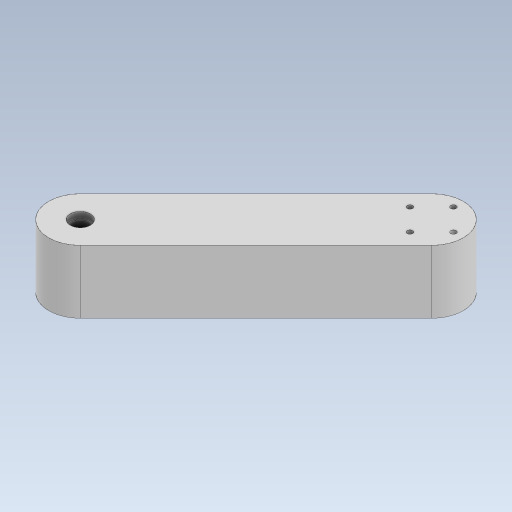
# Autodesk Inventor part: 5 Barras Simplificado
Saved by Autodesk Inventor 2024.2 (Build 282272000, 272)
## iProperties
Created: 2024-02-01
Part Number: 5 Barras Simplificado
Material: Generic
Document SubType Name: Modeling
Designer: juanp
Density: 1 g/cm^3
Appearance: Default
Author: juanp
Autodesk Inventor part; units mm, degrees
ref_plane "YZ Plane" through (0, 0, 0) normal (1, 0, 0) x (0, 1, 0)
ref_plane "XZ Plane" through (0, 0, 0) normal (0, 1, 0) x (-1, 0, 0)
ref_plane "XY Plane" through (0, 0, 0) normal (0, 0, 1) x (1, 0, 0)
sketch "Sketch1" plane through (0, 0, 0) normal (0, 1, 0) x (-1, 0, 0)
  line L0 (1000, 500) -> (0, 500) construction
  line L1 (0, 500) -> (0, -500) construction
  line L2 (0, -500) -> (1000, -500) construction
  line L3 (1000, -500) -> (1000, 500) construction
  line L4 (0, 75) -> (0, -75) construction
  line L5 (25.4, 75) -> (25.4, -75)
  line L6 (-25.4, -75) -> (-25.4, 75)
  arc A0 (25.4, 75) -> (-25.4, 75) centre (0, 75) ccw
  arc A1 (-25.4, -75) -> (25.4, -75) centre (0, -75) ccw
  line L7 (141.4214, 216.4214) -> (0, 75) construction
  line L8 (123.4608, 234.3819) -> (-17.9605, 92.9605)
  line L9 (17.9605, 57.0395) -> (159.3819, 198.4608)
  arc A2 (159.3819, 198.4608) -> (123.4608, 234.3819) centre (141.4214, 216.4214) ccw
  arc A3 (-17.9605, 92.9605) -> (17.9605, 57.0395) centre (0, 75) ccw
  line L10 (141.4214, -216.4214) -> (0, -75) construction
  line L11 (159.3819, -198.4608) -> (17.9605, -57.0395)
  line L12 (-17.9605, -92.9605) -> (123.4608, -234.3819)
  arc A4 (123.4608, -234.3819) -> (159.3819, -198.4608) centre (141.4214, -216.4214) ccw
  arc A5 (17.9605, -57.0395) -> (-17.9605, -92.9605) centre (0, -75) ccw
  line L13 (141.4214, 216.4214) -> (477.8167, 0) construction
  line L14 (155.1641, 237.7825) -> (491.5594, 21.3611)
  line L15 (464.0739, -21.3611) -> (127.6786, 195.0603)
  arc A6 (155.1641, 237.7825) -> (127.6786, 195.0603) centre (141.4214, 216.4214) ccw
  arc A7 (464.0739, -21.3611) -> (491.5594, 21.3611) centre (477.8167, 0) ccw
  line L16 (141.4214, -216.4214) -> (477.8167, 0) construction
  line L17 (155.1641, -237.7825) -> (491.5594, -21.3611)
  line L18 (464.0739, 21.3611) -> (127.6786, -195.0603)
  arc A8 (127.6786, -195.0603) -> (155.1641, -237.7825) centre (141.4214, -216.4214) ccw
  arc A9 (491.5594, -21.3611) -> (464.0739, 21.3611) centre (477.8167, 0) ccw
  line L19 (141.4214, -216.4214) -> (141.4214, -645.1752) construction
  line L20 (141.4214, 216.4214) -> (141.4214, 12.316) construction
  point P0 (0, 0)
  point P1 (0, 0)
  point P2 (0, 0)
  point P3 (70.7107, 145.7107)
  point P4 (70.7107, -145.7107)
  point P5 (309.619, 108.2107)
  point P6 (309.619, -108.2107)
  point P7 (-17.9605, 92.9605)
  point P8 (123.4608, -234.3819)
  point P9 (155.1641, -237.7825)
  point P10 (491.5594, -21.3611)
  point P11 (491.5594, 21.3611)
  point P12 (155.1641, 237.7825)
  point P13 (123.4608, 234.3819)
  point P14 (-25.4, -75)
  point P15 (-17.9605, -92.9605)
  dimension "d42" = 1000
  dimension "d43" = 1000
  dimension "d45" = 150
  dimension "d46" = 50.8
  dimension "d47" = 50.8
  dimension "d48" = 50.8
  dimension "d49" = 50.8
  dimension "d50" = 50.8
  dimension "d51" = 200
  dimension "d52" = 200
  dimension "d53" = 400
  dimension "d54" = 400
  dimension "d55" = 45
  dimension "d56" = 45
  dimension "d71" = 122.755
  dimension "d72" = 57.245
  dimension "d73" = 309.619
  dimension "d74" = 108.2107
  dimension "d75" = 70.7107
  dimension "d76" = 145.7107
  dimension "d77" = 77.755
  dimension "d78" = 75
  constraints: 52 end point, 20 point on circle, 20 tangent, 10 centre point, 7 parallel, 6 midpoint, 3 vertical, 2 coincident, 1 horizontal, 1 perpendicular
  measures "d42" distance of L2.end L1.end
  measures "d43" distance of L2.end L0.start
  measures "d45" distance of L4.start L4.end
  measures "d46" distance between parallel lines of L5 L6
  measures "d47" distance between parallel lines of L14 L15
  measures "d48" distance between parallel lines of L17 L18
  measures "d49" distance between parallel lines of L9 L8
  measures "d50" distance between parallel lines of L12 L11
  measures "d51" distance of L4.start L7.start
  measures "d52" distance of L4.end L10.start
  measures "d53" distance of L13.end L7.start
  measures "d54" distance of L10.start L13.end
  measures "d55" angle of L10 L4
  measures "d56" angle of L7 L1
  measures "d71" angle of L16 L19
  measures "d72" angle of L13 L20
  measures "d73" distance from line of point (309.619, -108.211) L1
  measures "d74" vertical distance of point (309.619, -108.211) point (0, 0)
  measures "d75" horizontal distance of point (70.711, -145.711) point (0, 0)
  measures "d76" vertical distance of point (70.711, -145.711) point (0, 0)
  measures "d77" angle of L13 L7
  measures "d78" distance of L4.start point (0, 0)
extrude "Extrusion6" add sketch "Sketch1" against normal blind 50.8 contours A0 L8 A6 L15 L9 L5 | L5 L9 A3 A0 | L15 A6 A2 L9
extrude "Extrusion7" add sketch "Sketch1" along normal blind 53.8 separate body contours L15 A6 A2 L9 | L9 A2 L14 A9 L18 L15 | L18 A9 A7 L15
extrude "Extrusion13" cut sketch "Sketch1" along normal blind 3 contours L15 A6 A2 L9 | L9 A2 L14 A9 L18 L15 | L18 A9 A7 L15 bodies 2
extrude "Extrusion8" add sketch "Sketch1" along normal blind 107.6 separate body contours L18 L15 A7 L17 A4 L11 | L11 A4 A8 L18 | L18 A9 A7 L15
extrude "Extrusion10" cut sketch "Sketch1" along normal blind 56.8 contours L18 L15 A7 L17 A4 L11 | L11 A4 A8 L18 | L18 A9 A7 L15 bodies 3
extrude "Extrusion9" add sketch "Sketch1" along normal blind 161.4 separate body contours L11 L18 A8 L12 A1 L5 | L5 A1 A5 L11 | L11 A4 A8 L18
extrude "Extrusion11" cut sketch "Sketch1" along normal blind 110.6 contours L11 L18 A8 L12 A1 L5 | L5 A1 A5 L11 | L11 A4 A8 L18 bodies 4
sketch "Sketch6" plane through (0, 0, 0) normal (0, 1, 0) x (1, 0, 0)
  arc A0 (17.9605, -92.9605) -> (-17.9605, -57.0395) centre (0, -75) ccw construction
  line L0 (0, -92.5) -> (-17.5, -75) construction
  line L1 (-17.5, -75) -> (0, -57.5) construction
  line L2 (0, -57.5) -> (17.5, -75) construction
  line L3 (17.5, -75) -> (0, -92.5) construction
  line L4 (0, -92.5) -> (0, -57.5) construction
  line L5 (-17.5, -75) -> (17.5, -75) construction
  circle A1 centre (0, -75) radius 17.5 construction
  line L6 (-123.4608, -234.3819) -> (17.9605, -92.9605) construction
  circle A2 centre (0, -92.5) radius 2.15
  circle A3 centre (-17.5, -75) radius 2.15
  circle A4 centre (17.5, -75) radius 2.15
  circle A5 centre (0, -57.5) radius 2.15
  arc A6 (-159.3819, -198.4608) -> (-123.4608, -234.3819) centre (-141.4214, -216.4214) ccw construction
  circle A7 centre (-141.4214, -216.4214) radius 8.075
  circle A8 centre (-141.4214, -216.4214) radius 7.075
  circle A9 centre (-141.4214, -216.4214) radius 7.875
  point P0 (0, 0)
  point P1 (0, -75)
  dimension "d83" = 35
  dimension "d84" = 4.3
  dimension "d87" = 16.15
  dimension "d90" = 1
  dimension "d96" = 0.2
  constraints: 12 end point, 9 coincident, 7 centre point, 3 equal radius, 3 parallel, 2 perpendicular, 1 horizontal alignment, 1 midpoint, 2 other
  measures "d84" diameter of A3
  measures "d87" diameter of A7
  measures "d90" radial gap between concentric circles of A7 A8
  measures "d96" radial gap between concentric circles of A9 A7
extrude "Extrusion14" cut sketch "Sketch6" against normal through all contours A2 | A3 | A4 | A5 bodies 1
extrude "Extrusion15" cut sketch "Sketch6" against normal through all contours A7 | A8 | A9 bodies 1
extrude "Extrusion17" add sketch "Sketch6" against normal blind 45.8 separate body contours A9
extrude "Extrusion18" cut sketch "Sketch6" against normal blind 5 contours A9 bodies 5
ref_plane "Work Plane2" through (0, -25.4, 0) normal (0, 1, 0) x (1, 0, 0)
ref_plane "Work Plane4" through (0, 1.5, 0) normal (0, -1, 0) x (1, 0, 0)
mirror "Mirror2" about plane through (0, 1.5, 0) normal (0, -1, 0) of "Extrusion15" bodies 1 2
ref_plane "Work Plane5" through (-127.6786, 3, 195.0603) normal (0.8409882, 0, 0.5410534) x (0, 1, 0)
ref_plane "Work Plane6" through (-491.5594, 53.8, 21.3611) normal (0.8409882, 0, 0.5410534) x (0, -1, 0)
equation "\"d45\" = L_G"
equation "\"d46\" = t"
equation "\"d47\" = t"
equation "\"d48\" = t"
equation "\"d49\" = t"
equation "\"d50\" = t"
equation "\"d51\" = L_P"
equation "\"d52\" = L_P"
equation "\"d53\" = L_D"
equation "\"d54\" = L_D"
equation "\"d57\" = t"
equation "\"d59\" = t + sep"
equation "\"d79\" = sep"
equation "\"d61\" = 2 * t + 2 * sep"
equation "\"L_G\" = 150 * scale"
equation "\"L_P\" = 200 * scale"
equation "\"L_D\" = 400 * scale"
equation "\"t\" = 50.8 * scale"
equation "\"sep\" = 3"
equation "\"scale\" = 1"
body "Solid6"
body "Solid7"
body "Solid8"
body "Solid9"
body "Solid12"
